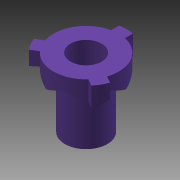
# Autodesk Inventor part: Rotor
Saved by Autodesk Inventor 2014 (Build 180170000, 170)
## iProperties
Created: 2017-02-07
Part Number: Rotor
Material: Generic
Document SubType Name: Modeling
Designer: Rubén
Density: 1 g/cm^3
Appearance: Violet
Author: Rubén
Autodesk Inventor part; units mm, degrees
ref_plane "YZ Plane" through (0, 0, 0) normal (1, 0, 0) x (0, 1, 0)
ref_plane "XZ Plane" through (0, 0, 0) normal (0, 1, 0) x (-1, 0, 0)
ref_plane "XY Plane" through (0, 0, 0) normal (0, 0, 1) x (1, 0, 0)
sketch "Sketch1" plane through (0, 0, 0) normal (0, 1, 0) x (-1, 0, 0)
  circle A0 centre (0, 0) radius 3.4
  dimension "d0" = 6.8
  constraints: 1 centre point, 1 coincident
  measures "d0" diameter of A0
extrude "Extrusion1" add sketch "Sketch1" along normal blind 9
sketch "Sketch2" plane through (0, 9, 0) normal (0, 1, 0) x (1, 0, 0)
  circle A0 centre (0, 0) radius 3.4 projected
  arc A1 (1.1, 6.4062) -> (-1.1, 6.4062) centre (0, 0) ccw
  line L0 (0, 6.5) -> (0, 0) construction
  line L1 (-1.1, 6.4062) -> (-1.1, 5.1335)
  line L2 (1.1, 6.4062) -> (1.1, 5.1335)
  arc A2 (1.1, 5.1335) -> (-1.1, 5.1335) centre (0, 0) ccw
  arc A3 (-6.098, -2.2505) -> (-4.998, -4.1558) centre (0, 0) ccw
  line L3 (-4.998, -4.1558) -> (-3.8957, -3.5194)
  line L4 (-6.098, -2.2505) -> (-4.9957, -1.6141)
  arc A4 (-4.9957, -1.6141) -> (-3.8957, -3.5194) centre (0, 0) ccw
  arc A5 (4.998, -4.1558) -> (6.098, -2.2505) centre (0, 0) ccw
  line L5 (6.098, -2.2505) -> (4.9957, -1.6141)
  line L6 (4.998, -4.1558) -> (3.8957, -3.5194)
  arc A6 (3.8957, -3.5194) -> (4.9957, -1.6141) centre (0, 0) ccw
  circle A7 centre (0, 0) radius 5.25
  point P0 (-5.6292, -3.25)
  point P1 (5.6292, -3.25)
  dimension "d19" = 10.5
  dimension "d3" = 2.2
  dimension "d8" = 6.5
  dimension "d17" = 360
  constraints: 14 end point, 13 point on circle, 6 centre point, 5 coincident, 2 parallel, 1 vertical, 37 other
  measures "d3" distance between parallel lines of L2 L1
  measures "d8" radius of A1
extrude "Extrusion2" add sketch "Sketch2" along normal blind 2 contours A0 | L2 A2 L1 A1 | A7 A6 A4 A2 | A4 L3 A3 L4 | L5 A5 L6 A6
sketch "Sketch4" plane through (0, 11, 0) normal (0, 1, 0) x (1, 0, 0)
  arc A0 (-6.098, -2.2505) -> (-4.998, -4.1558) centre (0, 0) ccw projected
hole "Hole2" at (0, 11, 0) direction (0, -1, 0) diameter 5 depth 6
sketch "Sketch5" plane through (0, 0, 0) normal (0, -1, 0) x (1, 0, 0)
  circle A0 centre (0, 0) radius 3.4 projected
  circle A1 centre (0, 0) radius 2.75
  dimension "d36" = 5.5
  constraints: 1 centre point, 1 coincident
  measures "d36" diameter of A1
hole "Hole3" at (0, 0, 0) direction (0, 1, 0) diameter 3 end through all counterbore diameter 6.2 counterbore depth 3
sketch "Sketch6" plane through (0, 9, 0) normal (0, -1, 0) x (1, 0, 0)
  arc A0 (-4.998, 4.1558) -> (-6.098, 2.2505) centre (0, 0) ccw projected
  line L0 (-4.9957, 1.6141) -> (-6.098, 2.2505) projected
  line L1 (-1.1, -6.4062) -> (-1.1, -5.1335) projected
  arc A1 (-1.1, -6.4062) -> (1.1, -6.4062) centre (0, 0) ccw projected
  line L2 (1.1, -5.1335) -> (1.1, -6.4062) projected
  line L3 (6.098, 2.2505) -> (4.9957, 1.6141) projected
  line L4 (3.8957, 3.5194) -> (4.998, 4.1558) projected
  arc A2 (3.8957, 3.5194) -> (-3.8957, 3.5194) centre (0, 0) ccw projected
  line L5 (-4.998, 4.1558) -> (-3.8957, 3.5194) projected
  circle A3 centre (0, 0) radius 3.4 projected
  line L6 (-3.7123, 3.7123) -> (0, 0) construction
  line L7 (-5.0711, 1.3588) -> (0, 0) construction
  line L8 (-5.0711, -1.3588) -> (0, 0) construction
  line L9 (-3.7123, -3.7123) -> (0, 0) construction
  line L10 (-1.3588, -5.0711) -> (0, 0) construction
  line L11 (1.3588, -5.0711) -> (0, 0) construction
  line L12 (3.7123, -3.7123) -> (0, 0) construction
  line L13 (5.0711, -1.3588) -> (0, 0) construction
  line L14 (5.0711, 1.3588) -> (0, 0) construction
  line L15 (3.7123, 3.7123) -> (0, 0) construction
  line L16 (1.3588, 5.0711) -> (0, 0) construction
  line L17 (-1.3588, 5.0711) -> (0, 0) construction
  line L18 (0, 0) -> (-5.6292, 3.25) construction
  line L19 (-3.7123, 3.7123) -> (-4.3917, 2.5356) construction
  line L20 (-4.3917, 2.5356) -> (-5.0711, 1.3588) construction
  line L21 (-3.7123, 3.7123) -> (-2.4042, 2.4042)
  line L22 (-5.0711, 1.3588) -> (-3.2841, 0.88)
  line L23 (-1.3588, 5.0711) -> (-0.88, 3.2841)
  line L24 (1.3588, 5.0711) -> (0.88, 3.2841)
  line L25 (3.7123, 3.7123) -> (2.4042, 2.4042)
  line L26 (5.0711, 1.3588) -> (3.2841, 0.88)
  line L27 (5.0711, -1.3588) -> (3.2841, -0.88)
  line L28 (3.7123, -3.7123) -> (2.4042, -2.4042)
  line L29 (1.3588, -5.0711) -> (0.88, -3.2841)
  line L30 (-1.3588, -5.0711) -> (-0.88, -3.2841)
  line L31 (-3.7123, -3.7123) -> (-2.4042, -2.4042)
  line L32 (-5.0711, -1.3588) -> (-3.2841, -0.88)
  arc A4 (-0.88, 3.2841) -> (-2.4042, 2.4042) centre (0, 0) ccw
  arc A5 (0.88, 3.2841) -> (-0.88, 3.2841) centre (0, 0) ccw
  arc A6 (2.4042, 2.4042) -> (0.88, 3.2841) centre (0, 0) ccw
  arc A7 (3.2841, 0.88) -> (2.4042, 2.4042) centre (0, 0) ccw
  arc A8 (3.2841, -0.88) -> (3.2841, 0.88) centre (0, 0) ccw
  arc A9 (2.4042, -2.4042) -> (3.2841, -0.88) centre (0, 0) ccw
  arc A10 (0.88, -3.2841) -> (2.4042, -2.4042) centre (0, 0) ccw
  arc A11 (-0.88, -3.2841) -> (0.88, -3.2841) centre (0, 0) ccw
  arc A12 (-2.4042, -2.4042) -> (-0.88, -3.2841) centre (0, 0) ccw
  arc A13 (-3.2841, -0.88) -> (-2.4042, -2.4042) centre (0, 0) ccw
  arc A14 (-3.2841, 0.88) -> (-3.2841, -0.88) centre (0, 0) ccw
  arc A15 (-2.4042, 2.4042) -> (-3.2841, 0.88) centre (0, 0) ccw
  arc A16 (-1.3588, 5.0711) -> (-3.7123, 3.7123) centre (0, 0) ccw
  arc A17 (1.3588, 5.0711) -> (-1.3588, 5.0711) centre (0, 0) ccw
  arc A18 (3.7123, 3.7123) -> (1.3588, 5.0711) centre (0, 0) ccw
  arc A19 (3.8957, 3.5194) -> (3.7123, 3.7123) centre (0, 0) ccw
  arc A20 (5.0711, 1.3588) -> (4.9957, 1.6141) centre (0, 0) ccw
  arc A21 (5.0711, -1.3588) -> (5.0711, 1.3588) centre (0, 0) ccw
  arc A22 (3.7123, -3.7123) -> (5.0711, -1.3588) centre (0, 0) ccw
  arc A23 (1.3588, -5.0711) -> (3.7123, -3.7123) centre (0, 0) ccw
  arc A24 (1.1, -5.1335) -> (1.3588, -5.0711) centre (0, 0) ccw
  arc A25 (-1.3588, -5.0711) -> (-1.1, -5.1335) centre (0, 0) ccw
  arc A26 (-3.7123, -3.7123) -> (-1.3588, -5.0711) centre (0, 0) ccw
  arc A27 (-5.0711, -1.3588) -> (-3.7123, -3.7123) centre (0, 0) ccw
  arc A28 (-5.0711, 1.3588) -> (-5.0711, -1.3588) centre (0, 0) ccw
  arc A29 (-4.9957, 1.6141) -> (-5.0711, 1.3588) centre (0, 0) ccw
  arc A30 (-3.7123, 3.7123) -> (-3.8957, 3.5194) centre (0, 0) ccw
  arc A31 (-4.998, 4.1558) -> (-6.098, 2.2505) centre (0, 0) ccw
  arc A32 (6.098, 2.2505) -> (4.998, 4.1558) centre (0, 0) ccw
  arc A33 (-1.1, -6.4062) -> (1.1, -6.4062) centre (0, 0) ccw
  line L33 (-1.1, -6.4062) -> (-1.1, -5.1335)
  line L34 (1.1, -6.4062) -> (1.1, -5.1335)
  line L35 (-6.098, 2.2505) -> (-4.9957, 1.6141)
  line L36 (-4.5466, 3.8952) -> (-3.8957, 3.5194)
  line L37 (4.998, 4.1558) -> (3.8957, 3.5194)
  line L38 (6.098, 2.2505) -> (4.9957, 1.6141)
  dimension "d46" = 360
  constraints: 66 end point, 62 point on circle, 30 centre point, 30 coincident, 14 point on line, 6 collinear, 1 parallel, 1 perpendicular, 50 other
extrude "Extrusion3" add sketch "Sketch6" along normal blind 1.2 contours L5 A2 L21 A3 L22 A29 L0 A0 | L32 A3 L31 A27 | A2 L24 A3 L23 | L30 A3 L29 A24 L2 A1 L1 A25 | A2 L4 A32 L3 A20 L26 A3 L25 | A3 L27 A22 L28
chamfer "Chamfer1" distance 1.2 angle 65 1 edges at (1.1194, 7.8, 4.1776) measured on face at (1.1194, 8.3, 4.1776)
chamfer "Chamfer2" distance 1.2 angle 65 1 edges at (4.1776, 7.8, 1.1194) measured on face at (4.1776, 8.3, 1.1194)
chamfer "Chamfer3" distance 1.2 angle 65 1 edges at (3.0582, 7.8, -3.0582) measured on face at (3.0582, 8.3, -3.0582)
chamfer "Chamfer4" distance 1.2 angle 65 1 edges at (-1.1194, 7.8, -4.1776) measured on face at (-1.1194, 8.3, -4.1776)
chamfer "Chamfer5" distance 1.2 angle 65 1 edges at (-4.1776, 7.8, -1.1194) measured on face at (-4.1776, 8.3, -1.1194)
chamfer "Chamfer6" distance 1.2 angle 65 1 edges at (-3.0582, 7.8, 3.0582) measured on face at (-3.0582, 8.3, 3.0582)
sketch "Sketch8" plane through (0, 9, 0) normal (0, -1, 0) x (1, 0, 0)
  line L0 (3.7123, -3.7123) -> (2.4042, -2.4042) projected
  arc A0 (0.88, -3.2841) -> (2.4042, -2.4042) centre (0, 0) ccw projected
  line L1 (0.88, -3.2841) -> (1.3588, -5.0711) projected
  arc A1 (1.3588, -5.0711) -> (3.7123, -3.7123) centre (0, 0) ccw projected
  line L2 (3.2841, -0.88) -> (5.0711, -1.3588) projected
  arc A2 (5.0711, -1.3588) -> (5.0711, 1.3588) centre (0, 0) ccw projected
  line L3 (5.0711, 1.3588) -> (3.2841, 0.88) projected
  arc A3 (3.2841, -0.88) -> (3.2841, 0.88) centre (0, 0) ccw projected
  line L4 (1.3588, 5.0711) -> (0.88, 3.2841) projected
  arc A4 (2.4042, 2.4042) -> (0.88, 3.2841) centre (0, 0) ccw projected
  line L5 (2.4042, 2.4042) -> (3.7123, 3.7123) projected
  arc A5 (3.7123, 3.7123) -> (1.3588, 5.0711) centre (0, 0) ccw projected
  line L6 (-0.88, 3.2841) -> (-1.3588, 5.0711) projected
  arc A6 (-1.3588, 5.0711) -> (-3.7123, 3.7123) centre (0, 0) ccw projected
  line L7 (-3.7123, 3.7123) -> (-2.4042, 2.4042) projected
  arc A7 (-0.88, 3.2841) -> (-2.4042, 2.4042) centre (0, 0) ccw projected
  line L8 (-3.2841, 0.88) -> (-5.0711, 1.3588) projected
  arc A8 (-5.0711, 1.3588) -> (-5.0711, -1.3588) centre (0, 0) ccw projected
  line L9 (-5.0711, -1.3588) -> (-3.2841, -0.88) projected
  arc A9 (-3.2841, 0.88) -> (-3.2841, -0.88) centre (0, 0) ccw projected
  line L10 (-1.3588, -5.0711) -> (-0.88, -3.2841) projected
  arc A10 (-2.4042, -2.4042) -> (-0.88, -3.2841) centre (0, 0) ccw projected
  line L11 (-2.4042, -2.4042) -> (-3.7123, -3.7123) projected
  arc A11 (-3.7123, -3.7123) -> (-1.3588, -5.0711) centre (0, 0) ccw projected
extrude "Extrusion5" add sketch "Sketch8" along normal blind 1.2
chamfer "Chamfer7" distance 1.2 angle 65 1 edges at (3.0582, 7.8, -3.0582) measured on face at (3.0582, 8.3, -3.0582)
chamfer "Chamfer8" distance 1.2 angle 65 1 edges at (-1.1194, 7.8, -4.1776) measured on face at (-1.1194, 8.3, -4.1776)
chamfer "Chamfer9" distance 1.2 angle 65 1 edges at (-4.1776, 7.8, -1.1194) measured on face at (-4.1776, 8.3, -1.1194)
chamfer "Chamfer10" distance 1.2 angle 65 1 edges at (-3.0582, 7.8, 3.0582) measured on face at (-3.0582, 8.3, 3.0582)
chamfer "Chamfer11" distance 1.2 angle 65 1 edges at (1.1194, 7.8, 4.1776) measured on face at (1.1194, 8.3, 4.1776)
chamfer "Chamfer12" distance 1.2 angle 65 1 edges at (4.1776, 7.8, 1.1194) measured on face at (4.1776, 8.3, 1.1194)
body "Solid1"
